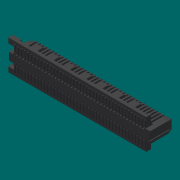
# Autodesk Inventor part: ST4-40-1.00-L-D-P-TR_terminal
Saved by Autodesk Inventor 2016 (Build 200138000, 138)
## iProperties
Category: PARTsolutions
Company: SAMTEC
Created: 2016-06-07
Part Number: ST4-40-1.00-L-D-P-TR_terminal
Catalog Web Link: www.cadenas.de
Description: ST4 Series Terminal-ST4 Series - (0,40 mm) .0158" Razor Beam™ LP Ultra Fine Pitch Header & Socket
Vendor: SAMTEC
Document SubType Name: Modeling
Designer: psAdmin
Manufacturer: SAMTEC
Mass: 0.0759161 g
Surface Area: 4.61206 cm^2
Volume: 0.0759161 cm^3
Density: 1 g/cm^3
Material: Generic
Appearance: PSOLRGB-127-127-127
PSOL_IDENT_0: {$CADENAS_DATA\23d-libs\samtec\modelling\st4\parts\st4_terminal.prj},241 {VTYP=3D},{NB=ST4-40-1.00-L
PSOL_IDENT_1: -D-P-TR_terminal},{LINA=ST4-40-1.00-L-D-P-TR_terminal},{NN=ST4 Series Terminal},{DATE=29.03.2016 09:
PSOL_IDENT_2: 31:56},{GEOMDATE=29.03.2016 09:31:00},{VERSION=},{LINEID=10},{LINESUBID=-1},{WBVAR=POS,LS,LOPT,POPT,
PSOL_IDENT_3: PAOPT,TROPT}  {NB=ST4-40-1.00-L-D-P-TR_terminal},{LINA=ST4-40-1.00-L-D-P-TR_terminal},{KT=DUMMY},{SE
PSOL_IDENT_4: RIES=ST4},{PN=ST4-40-1.00-L-D-P-TR},{POS=40},{POSATOF=40},{LS=1.00},{PLOPT=-L: 10micro\" Selective G
PSOL_IDENT_5: old in Contact Area, Matte Tin on Tail},{ROW=-D: Double},{LOPT=},{LOPTALG= '','Not Selected','L','-L
PSOL_IDENT_6: : Latching' },{LOPTPN=},{POPT=P},{POPTALG= '','Not Selected','P','-P: Pick & Place Pad' },{POPTPN=-P
PSOL_IDENT_7: },{PAOPT=},{PAOPTALG= '','Not Available' },{PAOPTPN=},{TROPT=TR},{TROPTALG= '','Not Selected','TR','
PSOL_IDENT_8: -TR: Tape & Reel' },{TROPTPN=-TR},{A=16.25},{B=15.6},{C=17.4},{F=22.46},{H=19.9},{J=19.5},{D=3.55},{
PSOL_IDENT_9: G=7.30},{K=0.00},{L=3.58},{DP=0.68000},{TP=2.76000},{PP=0.32000}
NN: ST4 Series Terminal
NT: ST4 Series - (0,40 mm) .0158" Razor Beam™ LP Ultra Fine Pitch Header & Socket
NB: ST4-40-1.00-L-D-P-TR_terminal
NBSYN: $PN._terminal
LINA: ST4-40-1.00-L-D-P-TR_terminal
SERIES: ST4
POS: 40
LS: 1.00
PLOPT: -L: 10micro" Selective Gold in Contact Area, Matte Tin on Tail
ROW: -D: Double
LOPT: Not Selected
POPT: -P: Pick & Place Pad
PAOPT: Not Available
TROPT: -TR: Tape & Reel
SUPPLIER: SAMTEC
ARTICLENO: ST4-40-1.00-L-D-P-TR_terminal
BOMINFO: ST4-40-1.00-L-D-P-TR_terminal
CREATOR: CADENAS GmbH
Title: ST4-40-1.00-L-D-P-TR_terminal
Author: Cadenas PARTsolutions
Comments: ST4 Series - (0,40 mm) .0158" Razor Beam™ LP Ultra Fine Pitch Header & Socket
Autodesk Inventor part; units mm, degrees
sketch "Sketch_2" plane through (0, 0.1, 0) normal (0, 1, 0) x (1, 0, 0)
  line L0 (-8.875, -1.225) -> (-8.875, -1.85)
  line L1 (-8.875, -1.85) -> (8.125, -1.85)
  line L2 (8.125, -1.85) -> (8.125, 1.85)
  line L3 (8.125, 1.85) -> (-8.875, 1.85)
  line L4 (-8.875, 1.85) -> (-8.875, 1.225)
  line L5 (-8.875, 1.225) -> (-8.125, 1.225)
  line L6 (-8.125, 1.225) -> (-8.125, -1.225)
  line L7 (-8.125, -1.225) -> (-8.875, -1.225)
  constraints: 16 end point
extrude "Extrusion1" add sketch "Sketch_2" along normal blind 0.58
sketch "Sketch_1" plane through (0, 0, 0) normal (0, 0, 1) x (1, 0, 0)
  line L0 (-8.695, 2.25) -> (-8.695, 0)
  line L1 (-8.695, 0) -> (8.705, 0)
  line L2 (8.705, 0) -> (8.705, 2.25)
  line L3 (8.705, 2.25) -> (-8.695, 2.25)
  constraints: 8 end point
extrude "Extrusion2" add sketch "Sketch_1" along normal mid plane 0.94
sketch "Sketch_4" plane through (-8.125, 0, 0) normal (1, 0, 0) x (0, 0, -1)
  line L0 (-0.68, 2.25) -> (-0.68, 0)
  line L1 (-0.68, 0) -> (0.68, 0)
  line L2 (0.68, 0) -> (0.68, 2.25)
  line L3 (0.68, 2.25) -> (0.5433, 2.76)
  line L4 (0.5433, 2.76) -> (-0.5433, 2.76)
  line L5 (-0.5433, 2.76) -> (-0.68, 2.25)
  constraints: 12 end point
extrude "Extrusion3" add sketch "Sketch_4" along normal blind 16.83
sketch "Sketch_3" plane through (0, 2.25, 0) normal (0, 1, 0) x (1, 0, 0)
  line L0 (-8.695, 0.47) -> (-8.695, -0.47)
  line L1 (-8.695, -0.47) -> (0.005, -0.47)
  line L2 (0.005, -0.47) -> (0.005, 0.47)
  line L3 (0.005, 0.47) -> (-8.695, 0.47)
  constraints: 8 end point
extrude "Extrusion4" add sketch "Sketch_3" along normal blind 0.51 draft -15
sketch "Sketch_5" plane through (0, 0, 0) normal (0, 0, 1) x (1, 0, 0)
  line L0 (8.4371, 3.25) -> (8.705, 2.25)
  line L1 (8.705, 2.25) -> (8.705, 3.25)
  line L2 (8.705, 3.25) -> (8.4371, 3.25)
  constraints: 6 end point
extrude "Extrusion5" cut sketch "Sketch_5" along normal mid plane 2.72
sketch "Sketch_6" plane through (0, 0, 0) normal (0, 1, 0) x (-1, 0, 0)
  line L0 (-8.605, 0.375) -> (-8.705, 0.375)
  line L1 (-8.705, 0.375) -> (-8.705, -0.375)
  line L2 (-8.705, -0.375) -> (-8.605, -0.375)
  line L3 (-8.605, -0.375) -> (-8.605, 0.375)
  constraints: 8 end point
extrude "Extrusion6" cut sketch "Sketch_6" along normal blind 5
sketch "Sketch_7" plane through (0, 0, 0) normal (1, 0, 0) x (0, 1, 0)
  line L0 (1.175, 1.85) -> (0.1, 1.85)
  line L1 (0.1, 1.85) -> (0.1, -1.85)
  line L2 (0.1, -1.85) -> (1.175, -1.85)
  line L3 (1.175, -1.85) -> (1.175, -1.65)
  line L4 (1.175, -1.65) -> (0.975, -1.55)
  line L5 (0.975, -1.55) -> (0.675, -1.55)
  line L6 (0.675, -1.55) -> (0.675, 1.55)
  line L7 (0.675, 1.55) -> (0.975, 1.55)
  line L8 (0.975, 1.55) -> (1.175, 1.65)
  line L9 (1.175, 1.65) -> (1.175, 1.85)
  constraints: 20 end point
extrude "Extrusion7" add sketch "Sketch_7" along normal mid plane 13.25
sketch "Sketch_8" plane through (0, 0, 0) normal (1, 0, 0) x (0, 1, 0)
  line L0 (0.68, 0.9765) -> (0.68, -0.9765)
  line L1 (0.68, -0.9765) -> (0.85, -0.8575)
  line L2 (0.85, -0.8575) -> (0.85, -0.78)
  arc A0 (0.95, -0.68) -> (0.85, -0.78) centre (0.95, -0.78) ccw
  line L3 (0.95, -0.68) -> (1, -0.68)
  line L4 (1, -0.68) -> (1, 0.68)
  line L5 (1, 0.68) -> (0.95, 0.68)
  arc A1 (0.85, 0.78) -> (0.95, 0.68) centre (0.95, 0.78) ccw
  line L6 (0.85, 0.78) -> (0.85, 0.8575)
  line L7 (0.85, 0.8575) -> (0.68, 0.9765)
  constraints: 16 end point, 4 point on circle, 2 centre point
extrude "Extrusion8" add sketch "Sketch_8" along normal mid plane 16.25
sketch "Sketch_9" plane through (0, 0.48, 0) normal (0, 1, 0) x (1, 0, 0)
  line L0 (-7.8005, -0.9765) -> (-7.8005, -1.85)
  line L1 (-7.8005, -1.85) -> (-6.3605, -1.85)
  line L2 (-6.3605, -1.85) -> (-6.3605, -1.4565)
  arc A0 (-6.2805, -1.3765) -> (-6.3605, -1.4565) centre (-6.2805, -1.4565) ccw
  arc A1 (-6.2805, -1.3765) -> (-6.2005, -1.2965) centre (-6.2805, -1.2965) ccw
  line L3 (-6.2005, -1.2965) -> (-6.2005, -0.9765)
  line L4 (-6.2005, -0.9765) -> (-7.8005, -0.9765)
  constraints: 10 end point, 4 point on circle, 2 centre point
extrude "Extrusion9" cut sketch "Sketch_9" along normal blind 1.2
sketch "Sketch_10" plane through (0, 0.48, 0) normal (0, 1, 0) x (1, 0, 0)
  line L0 (6.2005, -0.9765) -> (6.2005, -1.2965)
  arc A0 (6.2005, -1.2965) -> (6.2805, -1.3765) centre (6.2805, -1.2965) ccw
  arc A1 (6.3605, -1.4565) -> (6.2805, -1.3765) centre (6.2805, -1.4565) ccw
  line L1 (6.3605, -1.4565) -> (6.3605, -1.85)
  line L2 (6.3605, -1.85) -> (7.8005, -1.85)
  line L3 (7.8005, -1.85) -> (7.8005, -0.9765)
  line L4 (7.8005, -0.9765) -> (6.2005, -0.9765)
  constraints: 10 end point, 4 point on circle, 2 centre point
extrude "Extrusion10" cut sketch "Sketch_10" along normal blind 1.2
sketch "Sketch_11" plane through (0, 0.48, 0) normal (0, 1, 0) x (1, 0, 0)
  line L0 (-7.8005, 0.9765) -> (-6.2005, 0.9765)
  line L1 (-6.2005, 0.9765) -> (-6.2005, 1.2965)
  arc A0 (-6.2005, 1.2965) -> (-6.2805, 1.3765) centre (-6.2805, 1.2965) ccw
  arc A1 (-6.3605, 1.4565) -> (-6.2805, 1.3765) centre (-6.2805, 1.4565) ccw
  line L2 (-6.3605, 1.4565) -> (-6.3605, 1.85)
  line L3 (-6.3605, 1.85) -> (-7.8005, 1.85)
  line L4 (-7.8005, 1.85) -> (-7.8005, 0.9765)
  constraints: 10 end point, 4 point on circle, 2 centre point
extrude "Extrusion11" cut sketch "Sketch_11" along normal blind 1.2
sketch "Sketch_12" plane through (0, 0.48, 0) normal (0, 1, 0) x (1, 0, 0)
  line L0 (6.2005, 0.9765) -> (7.8005, 0.9765)
  line L1 (7.8005, 0.9765) -> (7.8005, 1.85)
  line L2 (7.8005, 1.85) -> (6.3605, 1.85)
  line L3 (6.3605, 1.85) -> (6.3605, 1.4565)
  arc A0 (6.2805, 1.3765) -> (6.3605, 1.4565) centre (6.2805, 1.4565) ccw
  arc A1 (6.2805, 1.3765) -> (6.2005, 1.2965) centre (6.2805, 1.2965) ccw
  line L4 (6.2005, 1.2965) -> (6.2005, 0.9765)
  constraints: 10 end point, 4 point on circle, 2 centre point
extrude "Extrusion12" cut sketch "Sketch_12" along normal blind 1.2
sketch "Sketch_15" plane through (0, 0.48, 0) normal (0, 1, 0) x (1, 0, 0)
  arc A0 (-5.8005, -1.2965) -> (-5.7205, -1.3765) centre (-5.7205, -1.2965) ccw
  arc A1 (-5.6405, -1.4565) -> (-5.7205, -1.3765) centre (-5.7205, -1.4565) ccw
  line L0 (-5.6405, -1.4565) -> (-5.6405, -2.85)
  line L1 (-5.6405, -2.85) -> (5.6405, -2.85)
  line L2 (5.6405, -2.85) -> (5.6405, -1.4565)
  arc A2 (5.7205, -1.3765) -> (5.6405, -1.4565) centre (5.7205, -1.4565) ccw
  arc A3 (5.7205, -1.3765) -> (5.8005, -1.2965) centre (5.7205, -1.2965) ccw
  line L3 (5.8005, -1.2965) -> (5.8005, -0.9765)
  line L4 (5.8005, -0.9765) -> (4.2005, -0.9765)
  line L5 (4.2005, -0.9765) -> (4.2005, -1.2965)
  arc A4 (4.2005, -1.2965) -> (4.2805, -1.3765) centre (4.2805, -1.2965) ccw
  arc A5 (4.3605, -1.4565) -> (4.2805, -1.3765) centre (4.2805, -1.4565) ccw
  line L6 (4.3605, -1.4565) -> (4.3605, -1.85)
  line L7 (4.3605, -1.85) -> (3.6395, -1.85)
  line L8 (3.6395, -1.85) -> (3.6395, -1.4565)
  arc A6 (3.7195, -1.3765) -> (3.6395, -1.4565) centre (3.7195, -1.4565) ccw
  arc A7 (3.7195, -1.3765) -> (3.7995, -1.2965) centre (3.7195, -1.2965) ccw
  line L9 (3.7995, -1.2965) -> (3.7995, -0.9765)
  line L10 (3.7995, -0.9765) -> (2.1995, -0.9765)
  line L11 (2.1995, -0.9765) -> (2.1995, -1.2965)
  arc A8 (2.1995, -1.2965) -> (2.2795, -1.3765) centre (2.2795, -1.2965) ccw
  arc A9 (2.3595, -1.4565) -> (2.2795, -1.3765) centre (2.2795, -1.4565) ccw
  line L12 (2.3595, -1.4565) -> (2.3595, -1.85)
  line L13 (2.3595, -1.85) -> (1.6395, -1.85)
  line L14 (1.6395, -1.85) -> (1.6395, -1.4565)
  arc A10 (1.7195, -1.3765) -> (1.6395, -1.4565) centre (1.7195, -1.4565) ccw
  arc A11 (1.7195, -1.3765) -> (1.7995, -1.2965) centre (1.7195, -1.2965) ccw
  line L15 (1.7995, -1.2965) -> (1.7995, -0.9765)
  line L16 (1.7995, -0.9765) -> (0.1995, -0.9765)
  line L17 (0.1995, -0.9765) -> (0.1995, -1.2965)
  arc A12 (0.1995, -1.2965) -> (0.2795, -1.3765) centre (0.2795, -1.2965) ccw
  arc A13 (0.3595, -1.4565) -> (0.2795, -1.3765) centre (0.2795, -1.4565) ccw
  line L18 (0.3595, -1.4565) -> (0.3595, -1.85)
  line L19 (0.3595, -1.85) -> (-0.3605, -1.85)
  line L20 (-0.3605, -1.85) -> (-0.3605, -1.4565)
  arc A14 (-0.2805, -1.3765) -> (-0.3605, -1.4565) centre (-0.2805, -1.4565) ccw
  arc A15 (-0.2805, -1.3765) -> (-0.2005, -1.2965) centre (-0.2805, -1.2965) ccw
  line L21 (-0.2005, -1.2965) -> (-0.2005, -0.9765)
  line L22 (-0.2005, -0.9765) -> (-1.8005, -0.9765)
  line L23 (-1.8005, -0.9765) -> (-1.8005, -1.2965)
  arc A16 (-1.8005, -1.2965) -> (-1.7205, -1.3765) centre (-1.7205, -1.2965) ccw
  arc A17 (-1.6405, -1.4565) -> (-1.7205, -1.3765) centre (-1.7205, -1.4565) ccw
  line L24 (-1.6405, -1.4565) -> (-1.6405, -1.85)
  line L25 (-1.6405, -1.85) -> (-2.3605, -1.85)
  line L26 (-2.3605, -1.85) -> (-2.3605, -1.4565)
  arc A18 (-2.2805, -1.3765) -> (-2.3605, -1.4565) centre (-2.2805, -1.4565) ccw
  arc A19 (-2.2805, -1.3765) -> (-2.2005, -1.2965) centre (-2.2805, -1.2965) ccw
  line L27 (-2.2005, -1.2965) -> (-2.2005, -0.9765)
  line L28 (-2.2005, -0.9765) -> (-3.8005, -0.9765)
  line L29 (-3.8005, -0.9765) -> (-3.8005, -1.2965)
  arc A20 (-3.8005, -1.2965) -> (-3.7205, -1.3765) centre (-3.7205, -1.2965) ccw
  arc A21 (-3.6405, -1.4565) -> (-3.7205, -1.3765) centre (-3.7205, -1.4565) ccw
  line L30 (-3.6405, -1.4565) -> (-3.6405, -1.85)
  line L31 (-3.6405, -1.85) -> (-4.3605, -1.85)
  line L32 (-4.3605, -1.85) -> (-4.3605, -1.4565)
  arc A22 (-4.2805, -1.3765) -> (-4.3605, -1.4565) centre (-4.2805, -1.4565) ccw
  arc A23 (-4.2805, -1.3765) -> (-4.2005, -1.2965) centre (-4.2805, -1.2965) ccw
  line L33 (-4.2005, -1.2965) -> (-4.2005, -0.9765)
  line L34 (-4.2005, -0.9765) -> (-5.8005, -0.9765)
  line L35 (-5.8005, -0.9765) -> (-5.8005, -1.2965)
  constraints: 72 end point, 48 point on circle, 24 centre point
extrude "Extrusion13" cut sketch "Sketch_15" along normal blind 1.2
sketch "Sketch_16" plane through (0, 0.48, 0) normal (0, 1, 0) x (1, 0, 0)
  line L0 (-5.8005, 1.2965) -> (-5.8005, 0.9765)
  line L1 (-5.8005, 0.9765) -> (-4.2005, 0.9765)
  line L2 (-4.2005, 0.9765) -> (-4.2005, 1.2965)
  arc A0 (-4.2005, 1.2965) -> (-4.2805, 1.3765) centre (-4.2805, 1.2965) ccw
  arc A1 (-4.3605, 1.4565) -> (-4.2805, 1.3765) centre (-4.2805, 1.4565) ccw
  line L3 (-4.3605, 1.4565) -> (-4.3605, 1.85)
  line L4 (-4.3605, 1.85) -> (-3.6405, 1.85)
  line L5 (-3.6405, 1.85) -> (-3.6405, 1.4565)
  arc A2 (-3.7205, 1.3765) -> (-3.6405, 1.4565) centre (-3.7205, 1.4565) ccw
  arc A3 (-3.7205, 1.3765) -> (-3.8005, 1.2965) centre (-3.7205, 1.2965) ccw
  line L6 (-3.8005, 1.2965) -> (-3.8005, 0.9765)
  line L7 (-3.8005, 0.9765) -> (-2.2005, 0.9765)
  line L8 (-2.2005, 0.9765) -> (-2.2005, 1.2965)
  arc A4 (-2.2005, 1.2965) -> (-2.2805, 1.3765) centre (-2.2805, 1.2965) ccw
  arc A5 (-2.3605, 1.4565) -> (-2.2805, 1.3765) centre (-2.2805, 1.4565) ccw
  line L9 (-2.3605, 1.4565) -> (-2.3605, 1.85)
  line L10 (-2.3605, 1.85) -> (-1.6405, 1.85)
  line L11 (-1.6405, 1.85) -> (-1.6405, 1.4565)
  arc A6 (-1.7205, 1.3765) -> (-1.6405, 1.4565) centre (-1.7205, 1.4565) ccw
  arc A7 (-1.7205, 1.3765) -> (-1.8005, 1.2965) centre (-1.7205, 1.2965) ccw
  line L12 (-1.8005, 1.2965) -> (-1.8005, 0.9765)
  line L13 (-1.8005, 0.9765) -> (-0.2005, 0.9765)
  line L14 (-0.2005, 0.9765) -> (-0.2005, 1.2965)
  arc A8 (-0.2005, 1.2965) -> (-0.2805, 1.3765) centre (-0.2805, 1.2965) ccw
  arc A9 (-0.3605, 1.4565) -> (-0.2805, 1.3765) centre (-0.2805, 1.4565) ccw
  line L15 (-0.3605, 1.4565) -> (-0.3605, 1.85)
  line L16 (-0.3605, 1.85) -> (0.3595, 1.85)
  line L17 (0.3595, 1.85) -> (0.3595, 1.4565)
  arc A10 (0.2795, 1.3765) -> (0.3595, 1.4565) centre (0.2795, 1.4565) ccw
  arc A11 (0.2795, 1.3765) -> (0.1995, 1.2965) centre (0.2795, 1.2965) ccw
  line L18 (0.1995, 1.2965) -> (0.1995, 0.9765)
  line L19 (0.1995, 0.9765) -> (1.7995, 0.9765)
  line L20 (1.7995, 0.9765) -> (1.7995, 1.2965)
  arc A12 (1.7995, 1.2965) -> (1.7195, 1.3765) centre (1.7195, 1.2965) ccw
  arc A13 (1.6395, 1.4565) -> (1.7195, 1.3765) centre (1.7195, 1.4565) ccw
  line L21 (1.6395, 1.4565) -> (1.6395, 1.85)
  line L22 (1.6395, 1.85) -> (2.3595, 1.85)
  line L23 (2.3595, 1.85) -> (2.3595, 1.4565)
  arc A14 (2.2795, 1.3765) -> (2.3595, 1.4565) centre (2.2795, 1.4565) ccw
  arc A15 (2.2795, 1.3765) -> (2.1995, 1.2965) centre (2.2795, 1.2965) ccw
  line L24 (2.1995, 1.2965) -> (2.1995, 0.9765)
  line L25 (2.1995, 0.9765) -> (3.7995, 0.9765)
  line L26 (3.7995, 0.9765) -> (3.7995, 1.2965)
  arc A16 (3.7995, 1.2965) -> (3.7195, 1.3765) centre (3.7195, 1.2965) ccw
  arc A17 (3.6395, 1.4565) -> (3.7195, 1.3765) centre (3.7195, 1.4565) ccw
  line L27 (3.6395, 1.4565) -> (3.6395, 1.85)
  line L28 (3.6395, 1.85) -> (4.3605, 1.85)
  line L29 (4.3605, 1.85) -> (4.3605, 1.4565)
  arc A18 (4.2805, 1.3765) -> (4.3605, 1.4565) centre (4.2805, 1.4565) ccw
  arc A19 (4.2805, 1.3765) -> (4.2005, 1.2965) centre (4.2805, 1.2965) ccw
  line L30 (4.2005, 1.2965) -> (4.2005, 0.9765)
  line L31 (4.2005, 0.9765) -> (5.8005, 0.9765)
  line L32 (5.8005, 0.9765) -> (5.8005, 1.2965)
  arc A20 (5.8005, 1.2965) -> (5.7205, 1.3765) centre (5.7205, 1.2965) ccw
  arc A21 (5.6405, 1.4565) -> (5.7205, 1.3765) centre (5.7205, 1.4565) ccw
  line L33 (5.6405, 1.4565) -> (5.6405, 2.85)
  line L34 (5.6405, 2.85) -> (-5.6405, 2.85)
  line L35 (-5.6405, 2.85) -> (-5.6405, 1.4565)
  arc A22 (-5.7205, 1.3765) -> (-5.6405, 1.4565) centre (-5.7205, 1.4565) ccw
  arc A23 (-5.7205, 1.3765) -> (-5.8005, 1.2965) centre (-5.7205, 1.2965) ccw
  constraints: 72 end point, 48 point on circle, 24 centre point
extrude "Extrusion14" cut sketch "Sketch_16" along normal blind 1.2
sketch "Sketch_19" plane through (0, 0, 0) normal (0, 1, 0) x (-1, 0, 0)
  line L0 (7.9125, 0.753) -> (7.6875, 0.753)
  line L1 (7.6875, 0.753) -> (7.6875, 0.465)
  line L2 (7.6875, 0.465) -> (7.9125, 0.465)
  line L3 (7.9125, 0.465) -> (7.9125, 0.753)
  constraints: 8 end point
extrude "Extrusion15" cut sketch "Sketch_19" along normal blind 5
pattern_linear "Rectangular Pattern1" count 40 spacing 0.4 along (1, 0, 0) count 2 spacing 1.218 along (0, 0, -1) of "Extrusion15"
sketch "Sketch_21" plane through (0, 0, 0) normal (0, 0, 1) x (1, 0, 0)
  circle A0 centre (-8.0275, 0.08) radius 0.08
  constraints: 1 centre point
extrude "Extrusion16" add sketch "Sketch_21" along normal mid plane 3
sketch "Pattern_4_SKETCH_1" plane through (0.4275, 0, 0) normal (0, 0, 1) x (1, 0, 0)
  circle A0 centre (-8.0275, 0.08) radius 0.08
  constraints: 1 centre point
sketch "Pattern_4_SKETCH_2" plane through (0.8275, 0, 0) normal (0, 0, 1) x (1, 0, 0)
  circle A0 centre (-8.0275, 0.08) radius 0.08
  constraints: 1 centre point
sketch "Pattern_4_SKETCH_3" plane through (1.2275, 0, 0) normal (0, 0, 1) x (1, 0, 0)
  circle A0 centre (-8.0275, 0.08) radius 0.08
  constraints: 1 centre point
sketch "Pattern_4_SKETCH_4" plane through (1.6275, 0, 0) normal (0, 0, 1) x (1, 0, 0)
  circle A0 centre (-8.0275, 0.08) radius 0.08
  constraints: 1 centre point
sketch "Pattern_4_SKETCH_5" plane through (2.0275, 0, 0) normal (0, 0, 1) x (1, 0, 0)
  circle A0 centre (-8.0275, 0.08) radius 0.08
  constraints: 1 centre point
sketch "Pattern_4_SKETCH_6" plane through (2.4275, 0, 0) normal (0, 0, 1) x (1, 0, 0)
  circle A0 centre (-8.0275, 0.08) radius 0.08
  constraints: 1 centre point
sketch "Pattern_4_SKETCH_7" plane through (2.8275, 0, 0) normal (0, 0, 1) x (1, 0, 0)
  circle A0 centre (-8.0275, 0.08) radius 0.08
  constraints: 1 centre point
sketch "Pattern_4_SKETCH_8" plane through (3.2275, 0, 0) normal (0, 0, 1) x (1, 0, 0)
  circle A0 centre (-8.0275, 0.08) radius 0.08
  constraints: 1 centre point
sketch "Pattern_4_SKETCH_9" plane through (3.6275, 0, 0) normal (0, 0, 1) x (1, 0, 0)
  circle A0 centre (-8.0275, 0.08) radius 0.08
  constraints: 1 centre point
sketch "Pattern_4_SKETCH_10" plane through (4.0275, 0, 0) normal (0, 0, 1) x (1, 0, 0)
  circle A0 centre (-8.0275, 0.08) radius 0.08
  constraints: 1 centre point
sketch "Pattern_4_SKETCH_11" plane through (4.4275, 0, 0) normal (0, 0, 1) x (1, 0, 0)
  circle A0 centre (-8.0275, 0.08) radius 0.08
  constraints: 1 centre point
sketch "Pattern_4_SKETCH_12" plane through (4.8275, 0, 0) normal (0, 0, 1) x (1, 0, 0)
  circle A0 centre (-8.0275, 0.08) radius 0.08
  constraints: 1 centre point
sketch "Pattern_4_SKETCH_13" plane through (5.2275, 0, 0) normal (0, 0, 1) x (1, 0, 0)
  circle A0 centre (-8.0275, 0.08) radius 0.08
  constraints: 1 centre point
sketch "Pattern_4_SKETCH_14" plane through (5.6275, 0, 0) normal (0, 0, 1) x (1, 0, 0)
  circle A0 centre (-8.0275, 0.08) radius 0.08
  constraints: 1 centre point
sketch "Pattern_4_SKETCH_15" plane through (6.0275, 0, 0) normal (0, 0, 1) x (1, 0, 0)
  circle A0 centre (-8.0275, 0.08) radius 0.08
  constraints: 1 centre point
sketch "Pattern_4_SKETCH_16" plane through (6.4275, 0, 0) normal (0, 0, 1) x (1, 0, 0)
  circle A0 centre (-8.0275, 0.08) radius 0.08
  constraints: 1 centre point
sketch "Pattern_4_SKETCH_17" plane through (6.8275, 0, 0) normal (0, 0, 1) x (1, 0, 0)
  circle A0 centre (-8.0275, 0.08) radius 0.08
  constraints: 1 centre point
sketch "Pattern_4_SKETCH_18" plane through (7.2275, 0, 0) normal (0, 0, 1) x (1, 0, 0)
  circle A0 centre (-8.0275, 0.08) radius 0.08
  constraints: 1 centre point
sketch "Pattern_4_SKETCH_19" plane through (7.6275, 0, 0) normal (0, 0, 1) x (1, 0, 0)
  circle A0 centre (-8.0275, 0.08) radius 0.08
  constraints: 1 centre point
sketch "Pattern_4_SKETCH_20" plane through (8.0275, 0, 0) normal (0, 0, 1) x (1, 0, 0)
  circle A0 centre (-8.0275, 0.08) radius 0.08
  constraints: 1 centre point
sketch "Pattern_4_SKETCH_21" plane through (8.4275, 0, 0) normal (0, 0, 1) x (1, 0, 0)
  circle A0 centre (-8.0275, 0.08) radius 0.08
  constraints: 1 centre point
sketch "Pattern_4_SKETCH_22" plane through (8.8275, 0, 0) normal (0, 0, 1) x (1, 0, 0)
  circle A0 centre (-8.0275, 0.08) radius 0.08
  constraints: 1 centre point
sketch "Pattern_4_SKETCH_23" plane through (9.2275, 0, 0) normal (0, 0, 1) x (1, 0, 0)
  circle A0 centre (-8.0275, 0.08) radius 0.08
  constraints: 1 centre point
sketch "Pattern_4_SKETCH_24" plane through (9.6275, 0, 0) normal (0, 0, 1) x (1, 0, 0)
  circle A0 centre (-8.0275, 0.08) radius 0.08
  constraints: 1 centre point
sketch "Pattern_4_SKETCH_25" plane through (10.0275, 0, 0) normal (0, 0, 1) x (1, 0, 0)
  circle A0 centre (-8.0275, 0.08) radius 0.08
  constraints: 1 centre point
sketch "Pattern_4_SKETCH_26" plane through (10.4275, 0, 0) normal (0, 0, 1) x (1, 0, 0)
  circle A0 centre (-8.0275, 0.08) radius 0.08
  constraints: 1 centre point
sketch "Pattern_4_SKETCH_27" plane through (10.8275, 0, 0) normal (0, 0, 1) x (1, 0, 0)
  circle A0 centre (-8.0275, 0.08) radius 0.08
  constraints: 1 centre point
sketch "Pattern_4_SKETCH_28" plane through (11.2275, 0, 0) normal (0, 0, 1) x (1, 0, 0)
  circle A0 centre (-8.0275, 0.08) radius 0.08
  constraints: 1 centre point
sketch "Pattern_4_SKETCH_29" plane through (11.6275, 0, 0) normal (0, 0, 1) x (1, 0, 0)
  circle A0 centre (-8.0275, 0.08) radius 0.08
  constraints: 1 centre point
sketch "Pattern_4_SKETCH_30" plane through (12.0275, 0, 0) normal (0, 0, 1) x (1, 0, 0)
  circle A0 centre (-8.0275, 0.08) radius 0.08
  constraints: 1 centre point
sketch "Pattern_4_SKETCH_31" plane through (12.4275, 0, 0) normal (0, 0, 1) x (1, 0, 0)
  circle A0 centre (-8.0275, 0.08) radius 0.08
  constraints: 1 centre point
sketch "Pattern_4_SKETCH_32" plane through (12.8275, 0, 0) normal (0, 0, 1) x (1, 0, 0)
  circle A0 centre (-8.0275, 0.08) radius 0.08
  constraints: 1 centre point
sketch "Pattern_4_SKETCH_33" plane through (13.2275, 0, 0) normal (0, 0, 1) x (1, 0, 0)
  circle A0 centre (-8.0275, 0.08) radius 0.08
  constraints: 1 centre point
sketch "Pattern_4_SKETCH_34" plane through (13.6275, 0, 0) normal (0, 0, 1) x (1, 0, 0)
  circle A0 centre (-8.0275, 0.08) radius 0.08
  constraints: 1 centre point
sketch "Pattern_4_SKETCH_35" plane through (14.0275, 0, 0) normal (0, 0, 1) x (1, 0, 0)
  circle A0 centre (-8.0275, 0.08) radius 0.08
  constraints: 1 centre point
sketch "Pattern_4_SKETCH_36" plane through (14.4275, 0, 0) normal (0, 0, 1) x (1, 0, 0)
  circle A0 centre (-8.0275, 0.08) radius 0.08
  constraints: 1 centre point
sketch "Pattern_4_SKETCH_37" plane through (14.8275, 0, 0) normal (0, 0, 1) x (1, 0, 0)
  circle A0 centre (-8.0275, 0.08) radius 0.08
  constraints: 1 centre point
sketch "Pattern_4_SKETCH_38" plane through (15.2275, 0, 0) normal (0, 0, 1) x (1, 0, 0)
  circle A0 centre (-8.0275, 0.08) radius 0.08
  constraints: 1 centre point
sketch "Pattern_4_SKETCH_39" plane through (15.6275, 0, 0) normal (0, 0, 1) x (1, 0, 0)
  circle A0 centre (-8.0275, 0.08) radius 0.08
  constraints: 1 centre point
sketch "Pattern_4_SKETCH_40" plane through (16.055, 0.0117, 0) normal (0, 0, 1) x (1, 0, 0)
  circle A0 centre (-8.0275, 0.08) radius 0.08
  constraints: 1 centre point
extrude "Extrusion17" add sketch "Pattern_4_SKETCH_1" along normal mid plane 3
extrude "Extrusion18" add sketch "Pattern_4_SKETCH_2" along normal mid plane 3
extrude "Extrusion19" add sketch "Pattern_4_SKETCH_3" along normal mid plane 3
extrude "Extrusion20" add sketch "Pattern_4_SKETCH_4" along normal mid plane 3
extrude "Extrusion21" add sketch "Pattern_4_SKETCH_5" along normal mid plane 3
extrude "Extrusion22" add sketch "Pattern_4_SKETCH_6" along normal mid plane 3
extrude "Extrusion23" add sketch "Pattern_4_SKETCH_7" along normal mid plane 3
extrude "Extrusion24" add sketch "Pattern_4_SKETCH_8" along normal mid plane 3
extrude "Extrusion25" add sketch "Pattern_4_SKETCH_9" along normal mid plane 3
extrude "Extrusion26" add sketch "Pattern_4_SKETCH_10" along normal mid plane 3
extrude "Extrusion27" add sketch "Pattern_4_SKETCH_11" along normal mid plane 3
extrude "Extrusion28" add sketch "Pattern_4_SKETCH_12" along normal mid plane 3
extrude "Extrusion29" add sketch "Pattern_4_SKETCH_13" along normal mid plane 3
extrude "Extrusion30" add sketch "Pattern_4_SKETCH_14" along normal mid plane 3
extrude "Extrusion31" add sketch "Pattern_4_SKETCH_15" along normal mid plane 3
extrude "Extrusion32" add sketch "Pattern_4_SKETCH_16" along normal mid plane 3
extrude "Extrusion33" add sketch "Pattern_4_SKETCH_17" along normal mid plane 3
extrude "Extrusion34" add sketch "Pattern_4_SKETCH_18" along normal mid plane 3
extrude "Extrusion35" add sketch "Pattern_4_SKETCH_19" along normal mid plane 3
extrude "Extrusion36" add sketch "Pattern_4_SKETCH_20" along normal mid plane 3
extrude "Extrusion37" add sketch "Pattern_4_SKETCH_21" along normal mid plane 3
extrude "Extrusion38" add sketch "Pattern_4_SKETCH_22" along normal mid plane 3
extrude "Extrusion39" add sketch "Pattern_4_SKETCH_23" along normal mid plane 3
extrude "Extrusion40" add sketch "Pattern_4_SKETCH_24" along normal mid plane 3
extrude "Extrusion41" add sketch "Pattern_4_SKETCH_25" along normal mid plane 3
extrude "Extrusion42" add sketch "Pattern_4_SKETCH_26" along normal mid plane 3
extrude "Extrusion43" add sketch "Pattern_4_SKETCH_27" along normal mid plane 3
extrude "Extrusion44" add sketch "Pattern_4_SKETCH_28" along normal mid plane 3
extrude "Extrusion45" add sketch "Pattern_4_SKETCH_29" along normal mid plane 3
extrude "Extrusion46" add sketch "Pattern_4_SKETCH_30" along normal mid plane 3
extrude "Extrusion47" add sketch "Pattern_4_SKETCH_31" along normal mid plane 3
extrude "Extrusion48" add sketch "Pattern_4_SKETCH_32" along normal mid plane 3
extrude "Extrusion49" add sketch "Pattern_4_SKETCH_33" along normal mid plane 3
extrude "Extrusion50" add sketch "Pattern_4_SKETCH_34" along normal mid plane 3
extrude "Extrusion51" add sketch "Pattern_4_SKETCH_35" along normal mid plane 3
extrude "Extrusion52" add sketch "Pattern_4_SKETCH_36" along normal mid plane 3
extrude "Extrusion53" add sketch "Pattern_4_SKETCH_37" along normal mid plane 3
extrude "Extrusion54" add sketch "Pattern_4_SKETCH_38" along normal mid plane 3
extrude "Extrusion55" add sketch "Pattern_4_SKETCH_39" along normal mid plane 3
extrude "Extrusion56" add sketch "Pattern_4_SKETCH_40" along normal mid plane 3
sketch "Sketch_23" plane through (0, 2.76, 0) normal (0, 1, 0) x (1, 0, 0)
  arc A0 (-7.8875, -0.1) -> (-7.7875, -0.2) centre (-7.7875, -0.1) ccw
  line L0 (-7.7875, -0.2) -> (-6.2466, -0.2)
  arc A1 (-6.2466, 0.2) -> (-6.2466, -0.2) centre (-6, 0) ccw
  line L1 (-6.2466, 0.2) -> (-7.7875, 0.2)
  arc A2 (-7.7875, 0.2) -> (-7.8875, 0.1) centre (-7.7875, 0.1) ccw
  line L2 (-7.8875, 0.1) -> (-7.8875, -0.1)
  constraints: 6 end point, 6 point on circle, 3 centre point
extrude "Extrusion57" cut sketch "Sketch_23" along normal mid plane 2.65
sketch "Sketch_25" plane through (0, 2.76, 0) normal (0, 1, 0) x (1, 0, 0)
  arc A0 (6.2466, -0.2) -> (6.2466, 0.2) centre (6, 0) ccw
  line L0 (6.2466, -0.2) -> (7.7875, -0.2)
  arc A1 (7.7875, -0.2) -> (7.8875, -0.1) centre (7.7875, -0.1) ccw
  line L1 (7.8875, -0.1) -> (7.8875, 0.1)
  arc A2 (7.8875, 0.1) -> (7.7875, 0.2) centre (7.7875, 0.1) ccw
  line L2 (7.7875, 0.2) -> (6.2466, 0.2)
  constraints: 6 end point, 6 point on circle, 3 centre point
extrude "Extrusion58" cut sketch "Sketch_25" along normal mid plane 2.65
sketch "Sketch_26" plane through (0, 2.76, 0) normal (0, 1, 0) x (1, 0, 0)
  arc A0 (-5.7534, -0.2) -> (-5.7534, 0.2) centre (-6, 0) ccw
  line L0 (-5.7534, -0.2) -> (-4.2466, -0.2)
  arc A1 (-4.2466, 0.2) -> (-4.2466, -0.2) centre (-4, 0) ccw
  line L1 (-4.2466, 0.2) -> (-5.7534, 0.2)
  constraints: 4 end point, 4 point on circle, 2 centre point
extrude "Extrusion59" cut sketch "Sketch_26" against normal blind 1.325
pattern_linear "Rectangular Pattern2" count 6 spacing 2 along (1, 0, 0) of "Extrusion59"
sketch "Sketch_28" plane through (0, 0.68, 0) normal (0, 1, 0) x (1, 0, 0)
  line L0 (-8.512, 1.85) -> (-8.262, 1.35)
  line L1 (-8.262, 1.35) -> (-8.012, 1.85)
  line L2 (-8.012, 1.85) -> (-8.512, 1.85)
  constraints: 6 end point
extrude "Extrusion60" cut sketch "Sketch_28" against normal blind 0.05
sketch "Sketch_51" plane through (-1.395, 0, 0) normal (1, 0, 0) x (0, 0, -1)
  line L0 (-2, 3.23) -> (-2, 2.76)
  line L1 (-2, 2.76) -> (-1.2618, 2.76)
  arc A0 (-1.112, 2.6178) -> (-1.2618, 2.76) centre (-1.2618, 2.61) ccw
  line L2 (-1.112, 2.6178) -> (-1.021, 0.871)
  line L3 (-1.021, 0.871) -> (-0.7751, 1.0999)
  arc A1 (-0.7751, 1.0999) -> (-0.789, 1.331) centre (-0.8773, 1.2097) ccw
  arc A2 (-0.851, 1.4449) -> (-0.789, 1.331) centre (-0.7012, 1.4527) ccw
  line L4 (-0.851, 1.4449) -> (-0.911, 2.6022)
  arc A3 (-0.7612, 2.76) -> (-0.911, 2.6022) centre (-0.7612, 2.61) ccw
  line L5 (-0.7612, 2.76) -> (0.7612, 2.76)
  arc A4 (0.911, 2.6022) -> (0.7612, 2.76) centre (0.7612, 2.61) ccw
  line L6 (0.911, 2.6022) -> (0.851, 1.4449)
  arc A5 (0.789, 1.331) -> (0.851, 1.4449) centre (0.7012, 1.4527) ccw
  arc A6 (0.789, 1.331) -> (0.7751, 1.0999) centre (0.8773, 1.2097) ccw
  line L7 (0.7751, 1.0999) -> (1.021, 0.871)
  line L8 (1.021, 0.871) -> (1.112, 2.6178)
  arc A7 (1.2618, 2.76) -> (1.112, 2.6178) centre (1.2618, 2.61) ccw
  line L9 (1.2618, 2.76) -> (2, 2.76)
  line L10 (2, 2.76) -> (2, 3.23)
  line L11 (2, 3.23) -> (-2, 3.23)
  constraints: 24 end point, 16 point on circle, 8 centre point
extrude "Extrusion61" [suppressed]
sketch "Sketch_52" plane through (0, 2.76, 0) normal (0, 1, 0) x (1, 0, 0)
  line L0 (-1.995, -0.5) -> (-1.395, -0.5)
  line L1 (-1.395, -0.5) -> (-1.395, 0.5)
  line L2 (-1.395, 0.5) -> (-1.995, 0.5)
  line L3 (-1.995, 0.5) -> (-1.995, -0.5)
  constraints: 8 end point
extrude "Extrusion62" [suppressed]
ref_plane "pin_XY" through (0, -0.32, 0) normal (0, 1, 0) x (1, 0, 0)
ref_plane "pin_YZ" through (0, -0.32, 0) normal (1, 0, 0) x (0, 0, -1)
ref_plane "pin_ZX" through (0, -0.32, 0) normal (0, 0, -1) x (0, 1, 0)
ref_plane "terminal_XY" through (0, 0, 0) normal (0, 1, 0) x (1, 0, 0)
ref_plane "terminal_YZ" through (0, 0, 0) normal (1, 0, 0) x (0, 0, -1)
ref_plane "terminal_ZX" through (0, 0, 0) normal (0, 0, -1) x (0, 1, 0)
body "Solid1"
